Autodesk Fusion 360 part; units mm, degrees
(part 2 of 2)
sketch "Sketch73" plane through (0, 0, 2.5) normal (0, 0, 1) x (-1, 0, 0)
  line L0 (-44.1, 40.6) -> (-45.1, 40.6)
  line L1 (-45.1, 40.6) -> (-45.1, 35.3)
  arc A0 (-45.1, 35.3) -> (-42.1, 32.3) centre (-42.1, 35.3) ccw
  line L2 (-42.1, 32.3) -> (43.1, 32.3)
  arc A1 (43.1, 32.3) -> (46.1, 35.3) centre (43.1, 35.3) ccw
  line L3 (46.1, 35.3) -> (46.1, 40.6)
  line L4 (46.1, 40.6) -> (45.1, 40.6)
  line L5 (45.1, 40.6) -> (45.1, 70.6)
  line L6 (45.1, 70.6) -> (46.1, 70.6)
  line L7 (46.1, 70.6) -> (46.1, 75.9)
  arc A2 (46.1, 75.9) -> (43.1, 78.9) centre (43.1, 75.9) ccw
  line L8 (43.1, 78.9) -> (-42.1, 78.9)
  arc A3 (-42.1, 78.9) -> (-45.1, 75.9) centre (-42.1, 75.9) ccw
  line L9 (-45.1, 75.9) -> (-45.1, 70.6)
  line L10 (-45.1, 70.6) -> (-44.1, 70.6)
  line L11 (-44.1, 70.6) -> (-44.1, 40.6)
  line L12 (-43.1, 43.6) -> (-43.1, 65.6)
  line L13 (-43.1, 65.6) -> (-42.1, 65.6)
  arc A4 (-41.1, 64.6) -> (-42.1, 65.6) centre (-42.1, 64.6) ccw
  line L14 (-41.1, 64.6) -> (-41.1, 44.6)
  arc A5 (-42.1, 43.6) -> (-41.1, 44.6) centre (-42.1, 44.6) ccw
  line L15 (-42.1, 43.6) -> (-43.1, 43.6)
  line L16 (44.1, 67.6) -> (44.1, 45.6)
  line L17 (44.1, 45.6) -> (43.1, 45.6)
  arc A6 (42.1, 46.6) -> (43.1, 45.6) centre (43.1, 46.6) ccw
  line L18 (42.1, 46.6) -> (42.1, 66.6)
  arc A7 (43.1, 67.6) -> (42.1, 66.6) centre (43.1, 66.6) ccw
  line L19 (43.1, 67.6) -> (44.1, 67.6)
  line L20 (44.3, 35.3) -> (44.3, 38.8)
  line L21 (44.3, 38.8) -> (43.3, 38.8)
  line L22 (43.3, 38.8) -> (43.3, 72.4)
  line L23 (43.3, 72.4) -> (44.3, 72.4)
  line L24 (44.3, 72.4) -> (44.3, 75.9)
  arc A8 (44.3, 75.9) -> (43.1, 77.1) centre (43.1, 75.9) ccw
  line L25 (43.1, 77.1) -> (-42.1, 77.1)
  arc A9 (-42.1, 77.1) -> (-43.3, 75.9) centre (-42.1, 75.9) ccw
  line L26 (-43.3, 75.9) -> (-43.3, 72.4)
  line L27 (-43.3, 72.4) -> (-42.3, 72.4)
  line L28 (-42.3, 72.4) -> (-42.3, 38.8)
  line L29 (-42.3, 38.8) -> (-43.3, 38.8)
  line L30 (-43.3, 38.8) -> (-43.3, 35.3)
  arc A10 (-43.3, 35.3) -> (-42.1, 34.1) centre (-42.1, 35.3) ccw
  line L31 (-42.1, 34.1) -> (43.1, 34.1)
  arc A11 (43.1, 34.1) -> (44.3, 35.3) centre (43.1, 35.3) ccw
  line L32 (44.3, 38.8) -> (43.3, 38.8)
  line L33 (44.3, 72.4) -> (42.3, 72.4)
  line L34 (42.3, 72.4) -> (42.3, 77.1)
  line L35 (42.3, 77.1) -> (42.3, 75.3)
  line L36 (42.3, 75.3) -> (44.3, 75.3)
  line L37 (-43.3, 72.4) -> (-41.3, 72.4)
  line L38 (44.3, 38.8) -> (42.3, 38.8)
  line L39 (42.3, 38.8) -> (42.3, 34.1)
  line L40 (42.3, 34.1) -> (42.3, 35.9)
  line L41 (42.3, 35.9) -> (44.3, 35.9)
  line L42 (-43.3, 38.8) -> (-41.3, 38.8)
  line L43 (-41.3, 38.8) -> (-41.3, 34.1)
  line L44 (-41.3, 34.1) -> (-41.3, 35.9)
  line L45 (-41.3, 35.9) -> (-43.3, 35.9)
  line L46 (-41.3, 72.4) -> (-41.3, 77.1)
  line L47 (-41.3, 77.1) -> (-41.3, 75.3)
  line L48 (-41.3, 75.3) -> (-43.3, 75.3)
  dimension "d275" = -1.8
  dimension "d278" = 2
  dimension "d279" = 1.8
  dimension "d280" = 2
  dimension "d281" = 2
  dimension "d282" = 1.8
  dimension "d283" = 180
  dimension "d284" = 2
  dimension "d285" = 1.8
  dimension "d286" = 1.8
  constraint perpendicular L18 L32
  constraint perpendicular L24 L33
  constraint coincident L25 L34.end
  constraint perpendicular L25 L34
  constraint perpendicular L25 L35
  constraint coincident L24 L36.end
  constraint perpendicular L24 L36
  constraint perpendicular L28 L37
  constraint perpendicular L22 L38
  constraint coincident L31 L39.end
  constraint perpendicular L31 L39
  constraint coincident L39 L40.end
  constraint coincident L20 L41.end
  constraint perpendicular L20 L41
  constraint coincident L31 L43.end
  constraint perpendicular L31 L43
  constraint vertical L44
  constraint coincident L30 L45.end
  constraint perpendicular L30 L45
  constraint coincident L25 L46.end
  constraint perpendicular L25 L46
  constraint perpendicular L37 L47
  constraint coincident L26 L48.end
  constraint perpendicular L26 L48
  measures "d278" distance of L23.end L33.end
  measures "d279" distance of L34.end L35.end
  measures "d280" distance of L26.end L37.end
  measures "d281" distance of L20.end L38.end
  measures "d282" distance of L39.end L40.end
  measures "d283" angle of L41 L42
  measures "d284" distance of L29.end L42.end
  measures "d285" distance of L43.end L44.end
  measures "d286" distance of L46.end L47.end
extrude "Extrude43" add sketch "Sketch73" along normal blind 2 contours L30 A10 L31 L43 L44 L45 | L25 A9 L26 L46 L47 L48 | L20 L31 A11 L39 L40 L41 | L24 A8 L25 L34 L35 L36 bodies 3
fillet "Fillet11" radius 0.4 12 edges at (-44.3, -35.9, 3.5) (-42.3, -35.9, 3.5) (-42.3, -34.1, 3.5) (-42.3, -77.1, 3.5) (-42.3, -75.3, 3.5) (-44.3, -75.3, 3.5) (41.3, -35.9, 3.5) (43.3, -35.9, 3.5) (41.3, -34.1, 3.5) (41.3, -77.1, 3.5) (41.3, -75.3, 3.5) (43.3, -75.3, 3.5) on bodies 3
sketch "Sketch74" plane through (0, 0, 0) normal (0, 0, -1) x (1, 0, 0)
  line L0 (38.15, 41.2) -> (37.3598, 44.5622)
  line L1 (37.3598, 44.5622) -> (39.189, 43.9549)
  line L2 (39.189, 43.9549) -> (38.4793, 40.9048)
  line L3 (38.4793, 40.9048) -> (38.15, 41.2)
  line L4 (37.4517, 44.839) -> (37.7923, 48.7439)
  line L5 (37.7923, 48.7439) -> (39.35, 44.5)
  line L6 (39.35, 44.5) -> (39.2554, 44.2401)
  line L7 (39.2554, 44.2401) -> (37.4517, 44.839)
  line L8 (41.1421, 38.0836) -> (38.6549, 40.3311)
  line L9 (38.6549, 40.3311) -> (39.4312, 43.6665)
  line L10 (39.4312, 43.6665) -> (41.1421, 38.0836)
  line L11 (36.8902, 43.1477) -> (37.1351, 41.7415)
  line L12 (37.1351, 41.7415) -> (34.6232, 41.7415)
  line L13 (34.6232, 41.7415) -> (32.75, 36.1)
  line L14 (32.75, 36.1) -> (30.5, 36.1)
  line L15 (30.5, 36.1) -> (35.102, 48.7439)
  line L16 (35.102, 48.7439) -> (36.9483, 48.7439)
  line L17 (36.9483, 48.7439) -> (35.0902, 43.1477)
  line L18 (35.0902, 43.1477) -> (36.8902, 43.1477)
  line L19 (38.8305, 39.7574) -> (41.3179, 37.5099)
  line L20 (41.3179, 37.5099) -> (41.75, 36.1)
  line L21 (41.75, 36.1) -> (39.95, 36.1)
  line L22 (39.95, 36.1) -> (38.8305, 39.7574)
  line L23 (-43.1, 34.3) -> (42.1, 34.3)
  arc A0 (42.1, 34.3) -> (43.1, 35.3) centre (42.1, 35.3) ccw
  line L24 (43.1, 35.3) -> (43.1, 75.9)
  arc A1 (43.1, 75.9) -> (42.1, 76.9) centre (42.1, 75.9) ccw
  line L25 (42.1, 76.9) -> (-43.1, 76.9)
  arc A2 (-43.1, 76.9) -> (-44.1, 75.9) centre (-43.1, 75.9) ccw
  line L26 (-44.1, 75.9) -> (-44.1, 35.3)
  arc A3 (-44.1, 35.3) -> (-43.1, 34.3) centre (-43.1, 35.3) ccw
  line L27 (-36.5, 70) -> (-37.5, 70)
  line L28 (-40, 70) -> (-41, 70)
  line L29 (-27, 70) -> (-28, 70)
  line L30 (-30.5, 70) -> (-31.5, 70)
  spline S0 degree 5 poles (-42, 67) (-41.68, 67.0758) (-41.04, 67.2209) (-40.08, 67.4187) (-38.8, 67.6419) (-37.2, 67.8491) (-35.6, 67.9779) (-34, 68.022) (-32.4, 67.9779) (-30.8, 67.8491) (-29.2, 67.6419) (-27.92, 67.4187) (-26.96, 67.2209) (-26.32, 67.0758) (-26, 67) knots 0 0 0 0 0 0 0.1 0.2 0.3 0.4 0.5 0.6 0.7 0.8 0.9 1 1 1 1 1 1
  spline S1 degree 5 poles (-42, 65.5) (-41.6829, 65.5756) (-41.0464, 65.7201) (-40.0852, 65.9173) (-38.7902, 66.1401) (-37.1481, 66.3474) (-35.4809, 66.4771) (-33.7872, 66.5227) (-32.0675, 66.4811) (-30.3251, 66.355) (-28.5641, 66.1495) (-27.1439, 65.9254) (-26.0737, 65.7251) (-25.3583, 65.5774) (-25, 65.5) knots 0 0 0 0 0 0 0.1 0.2 0.3 0.4 0.5 0.6 0.7 0.8 0.9 1 1 1 1 1 1
  line L31 (-42, 67) -> (-42, 65.5)
  spline S2 degree 5 poles (-24.5, 74.5) (-24.4383, 74.4328) (-24.3171, 74.2898) (-24.1419, 74.0492) (-23.9216, 73.6755) (-23.6734, 73.1137) (-23.4641, 72.4471) (-23.3158, 71.6637) (-23.2636, 70.7525) (-23.3511, 69.7006) (-23.6271, 68.4931) (-24.037, 67.3897) (-24.4682, 66.4783) (-24.8132, 65.8325) (-25, 65.5) knots 0 0 0 0 0 0 0.1 0.2 0.3 0.4 0.5 0.6 0.7 0.8 0.9 1 1 1 1 1 1
  line L32 (-24.1819, 66.9558) -> (-25.8181, 64.0442)
  spline S3 degree 5 poles (-26, 74.5) (-25.9034, 74.3618) (-25.7186, 74.0843) (-25.4671, 73.665) (-25.1837, 73.0996) (-24.922, 72.3815) (-24.7607, 71.6512) (-24.7076, 70.9077) (-24.766, 70.1506) (-24.9305, 69.3805) (-25.1927, 68.5985) (-25.474, 67.9642) (-25.7226, 67.4839) (-25.9048, 67.1616) (-26, 67) knots 0 0 0 0 0 0 0.1 0.2 0.3 0.4 0.5 0.6 0.7 0.8 0.9 1 1 1 1 1 1
  line L33 (-26, 74.5) -> (-24.5, 74.5)
  line L34 (-26.7275, 65.8732) -> (-23.2725, 65.1268)
  line L35 (-38.75, 74.5) -> (-41.5, 70)
  line L36 (-41.5, 70) -> (-40.5, 70)
  line L37 (-38.75, 74.5) -> (-36, 70)
  line L38 (-36, 70) -> (-37.5, 70)
  line L39 (-29.25, 74.5) -> (-32, 70)
  line L40 (-32, 70) -> (-30.5, 70)
  line L41 (-28, 70) -> (-26.5, 70)
  line L42 (-26.5, 70) -> (-29.25, 74.5)
  line L43 (-30.5, 70) -> (-29.2225, 72.0905)
  line L44 (-28, 70) -> (-29.2225, 72.0905)
  line L45 (-40, 70) -> (-38.75, 72.0455)
  line L46 (-37.5, 70) -> (-38.75, 72.0455)
  point P0 (-34, 68)
  point P1 (-34, 66.5)
  point P2 (-23.5, 72.5)
  point P3 (-24.7358, 70.9878)
  constraint parallel L27 L28
  constraint horizontal L29
  constraint parallel L29 L30
  constraint vertical L31
  constraint midpoint S1.end L32
  constraint horizontal L33
  constraint midpoint S1.end L34
  constraint horizontal L36
  constraint parallel L29 L41
  constraint parallel L39 L43
  constraint parallel L35 L45
extrude "Extrude44" cut sketch "Sketch74" against normal blind 0.8 contours L27 L28 L35 L36 L37 L38 L45 L46 | L29 L30 L39 L40 L41 L42 L43 L44 | S0 S1 L31 S2 S3 L33 bodies 3
extrude "Extrude45" cut 3 faces at (-39.6667, -72.1818, 0.8) (-38.4185, -67.0868, 0.8) (-30.1575, -72.1968, 0.8) along direction (0, 0, 1) blind 0.8 on bodies 3 bodies 3
move_body "Move12" bodies 3 to x (1, 0, 0) y (0, -1, 0) z (0, 0, -1) at (0, -56.8, 18)
sketch "Sketch75" plane through (0, 0, 18) normal (0, 0, 1) x (-1, 0, 0)
  line L0 (40, -13.2) -> (41.5, -13.2)
  line L1 (41.5, -13.2) -> (38.75, -17.7)
  line L2 (38.75, -17.7) -> (36, -13.2)
  line L3 (36, -13.2) -> (37.5, -13.2)
  line L4 (37.5, -13.2) -> (38.75, -15.2455)
  line L5 (38.75, -15.2455) -> (40, -13.2)
  line L6 (29.25, -17.7) -> (26.5, -13.2)
  line L7 (26.5, -13.2) -> (28, -13.2)
  line L8 (28, -13.2) -> (29.2225, -15.2905)
  line L9 (29.2225, -15.2905) -> (30.5, -13.2)
  line L10 (30.5, -13.2) -> (32, -13.2)
  line L11 (32, -13.2) -> (29.25, -17.7)
  spline S0 degree 5 poles (25, -8.7) (25.3583, -8.7774) (26.0737, -8.9251) (27.1439, -9.1254) (28.5641, -9.3495) (30.3251, -9.555) (32.0675, -9.6811) (33.7872, -9.7227) (35.4809, -9.6771) (37.1481, -9.5474) (38.7902, -9.3401) (40.0852, -9.1173) (41.0464, -8.9201) (41.6829, -8.7756) (42, -8.7) knots -1 -1 -1 -1 -1 -1 -0.9 -0.8 -0.7 -0.6 -0.5 -0.4 -0.3 -0.2 -0.1 0 0 0 0 0 0
  line L12 (42, -8.7) -> (42, -10.2)
  spline S1 degree 5 poles (42, -10.2) (41.68, -10.2758) (41.04, -10.4209) (40.08, -10.6187) (38.8, -10.8419) (37.2, -11.0491) (35.6, -11.1779) (34, -11.222) (32.4, -11.1779) (30.8, -11.0491) (29.2, -10.8419) (27.92, -10.6187) (26.96, -10.4209) (26.32, -10.2758) (26, -10.2) knots 0 0 0 0 0 0 0.1 0.2 0.3 0.4 0.5 0.6 0.7 0.8 0.9 1 1 1 1 1 1
  spline S2 degree 5 poles (26, -10.2) (25.9048, -10.3616) (25.7226, -10.6839) (25.474, -11.1642) (25.1927, -11.7985) (24.9305, -12.5805) (24.766, -13.3506) (24.7076, -14.1077) (24.7607, -14.8512) (24.922, -15.5815) (25.1837, -16.2996) (25.4671, -16.865) (25.7186, -17.2843) (25.9034, -17.5618) (26, -17.7) knots -1 -1 -1 -1 -1 -1 -0.9 -0.8 -0.7 -0.6 -0.5 -0.4 -0.3 -0.2 -0.1 0 0 0 0 0 0
  line L13 (26, -17.7) -> (24.5, -17.7)
  spline S3 degree 5 poles (24.5, -17.7) (24.4383, -17.6328) (24.3171, -17.4898) (24.1419, -17.2492) (23.9216, -16.8755) (23.6734, -16.3137) (23.4641, -15.6471) (23.3158, -14.8637) (23.2636, -13.9525) (23.3511, -12.9006) (23.6271, -11.6931) (24.037, -10.5897) (24.4682, -9.6783) (24.8132, -9.0325) (25, -8.7) knots 0 0 0 0 0 0 0.1 0.2 0.3 0.4 0.5 0.6 0.7 0.8 0.9 1 1 1 1 1 1
  line L14 (-38.15, 15.6) -> (-37.3598, 12.2378)
  line L15 (-37.3598, 12.2378) -> (-39.189, 12.8451)
  line L16 (-39.189, 12.8451) -> (-38.4793, 15.8952)
  line L17 (-38.4793, 15.8952) -> (-38.15, 15.6)
  line L18 (-37.4517, 11.961) -> (-37.7923, 8.0561)
  line L19 (-37.7923, 8.0561) -> (-39.35, 12.3)
  line L20 (-39.35, 12.3) -> (-39.2554, 12.5599)
  line L21 (-39.2554, 12.5599) -> (-37.4517, 11.961)
  line L22 (-41.1421, 18.7164) -> (-38.6549, 16.4689)
  line L23 (-38.6549, 16.4689) -> (-39.4312, 13.1335)
  line L24 (-39.4312, 13.1335) -> (-41.1421, 18.7164)
  line L25 (-36.8902, 13.6523) -> (-37.1351, 15.0585)
  line L26 (-37.1351, 15.0585) -> (-34.6232, 15.0585)
  line L27 (-34.6232, 15.0585) -> (-32.75, 20.7)
  line L28 (-32.75, 20.7) -> (-30.5, 20.7)
  line L29 (-30.5, 20.7) -> (-35.102, 8.0561)
  line L30 (-35.102, 8.0561) -> (-36.9483, 8.0561)
  line L31 (-36.9483, 8.0561) -> (-35.0902, 13.6523)
  line L32 (-35.0902, 13.6523) -> (-36.8902, 13.6523)
  line L33 (-38.8305, 17.0426) -> (-41.3179, 19.2901)
  line L34 (-41.3179, 19.2901) -> (-41.75, 20.7)
  line L35 (-41.75, 20.7) -> (-39.95, 20.7)
  line L36 (-39.95, 20.7) -> (-38.8305, 17.0426)
  line L37 (43.1, 22.5) -> (-42.1, 22.5)
  arc A0 (-42.1, 22.5) -> (-43.1, 21.5) centre (-42.1, 21.5) ccw
  line L38 (-43.1, 21.5) -> (-43.1, -19.1)
  arc A1 (-43.1, -19.1) -> (-42.1, -20.1) centre (-42.1, -19.1) ccw
  line L39 (-42.1, -20.1) -> (43.1, -20.1)
  arc A2 (43.1, -20.1) -> (44.1, -19.1) centre (43.1, -19.1) ccw
  line L40 (44.1, -19.1) -> (44.1, 21.5)
  arc A3 (44.1, 21.5) -> (43.1, 22.5) centre (43.1, 21.5) ccw
  line L41 (-3, 16.7508) -> (-3, 11)
  line L42 (-3, 11) -> (-5, 11)
  line L43 (-5, 11) -> (-3.7917, 16.8319)
  line L44 (-6, 11) -> (-8, 11)
  arc A4 (-3, 16.7508) -> (-3.7917, 16.8319) centre (-3.4, 16.7508) ccw
  line L45 (-6, 11) -> (-6, 15.7508)
  line L46 (-8, 11) -> (-6.7881, 15.8478)
  arc A5 (-6, 15.7508) -> (-6.7881, 15.8478) centre (-6.4, 15.7508) ccw
  line L47 (-11.0916, 11.0065) -> (-8.9686, 11.0061)
  line L48 (-8.9686, 11.0061) -> (-8.967, 18.2622)
  line L49 (-9.7605, 18.3337) -> (-11.0916, 11.0065)
  arc A6 (-8.967, 18.2622) -> (-9.7605, 18.3337) centre (-9.367, 18.2622) ccw
  dimension "d295" = 0.4
  dimension "d299" = 0.4
  dimension "d304" = 0.4
  constraint perpendicular L41 L42
  constraint tangent L41 A4
  constraint tangent L43 A4
  constraint perpendicular L44 L45
  constraint tangent L45 A5
  constraint tangent L46 A5
  constraint perpendicular L47 L48
  constraint tangent L48 A6
  constraint tangent L49 A6
  measures "d295" radius of A4
  measures "d299" radius of A5
  measures "d304" radius of A6
extrude "Extrude46" cut sketch "Sketch75" against normal blind 3 contours L41 L42 L43 A4 | L44 L45 L46 A5 | L47 L48 L49 A6 bodies 3
move_body "Move14" bodies 3 to x (1, 0, 0) y (0, -1, 0) z (0, 0, -1) at (0, -59, 25)
move_body "Move15" bodies 3 to x (1, 0, 0) y (0, 1, 0) z (0, 0, 1) at (0, 0, -10)
move_body "Move16" bodies 3 to x (1, 0, 0) y (0, 1, 0) z (0, 0, 1) at (0, 0, 3)
component "Component" placed x (1, 0, 0) y (0, 1, 0) z (0, 0, 1) at (0, 0, 0)
component "Component" placed x (-1, 0, 0) y (0, -1, 0) z (0, 0, 1) at (-12, 0, 0)
